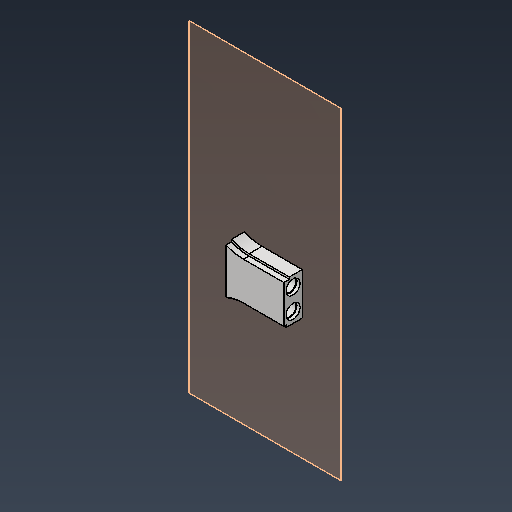
# Autodesk Inventor part: BearigHold
Saved by Autodesk Inventor 2026.2 (Build 302298010, 298A)
## iProperties
Created: 2026-04-04
Part Number: BearigHold
Material: Generic
Document SubType Name: Modeling
Designer: szymo
Density: 1 g/cm^3
Appearance: Default
Author: szymo
Autodesk Inventor part; units mm, degrees
ref_plane "YZ Plane" through (0, 0, 0) normal (1, 0, 0) x (0, 1, 0)
ref_plane "XZ Plane" through (0, 0, 0) normal (0, 1, 0) x (-1, 0, 0)
ref_plane "XY Plane" through (0, 0, 0) normal (0, 0, 1) x (1, 0, 0)
ref_plane "Work Plane1" through (11.7, -32.6479, 0) normal (0, 0, 1) x (-1, 0, 0)
sketch "Sketch1" plane through (11.7, -32.6479, 0) normal (0, 0, 1) x (-1, 0, 0)
  circle A0 centre (14.5, -14.5) radius 13.85 projected
  circle A1 centre (14.5, -14.5) radius 14.5 projected
  circle A2 centre (14.5, -55.2958) radius 13.85 projected
  circle A3 centre (14.5, -55.2958) radius 14.5 projected
  circle A4 centre (13, -35.0012) radius 5 projected
  line L0 (0, 0) -> (33.1738, 0)
  line L1 (33.1738, 0) -> (33.1738, -67)
  line L2 (33.1738, -67) -> (0, -67)
  line L3 (0, -67) -> (0, 0)
  line L4 (2, 0) -> (2, -67)
  line L5 (14.5, -28.35) -> (2, -28.35)
  line L6 (14.5, -29) -> (2, -29)
  line L7 (14.5, -40.7958) -> (2, -40.7958)
  line L8 (14.5, -41.4458) -> (2, -41.4458)
  line L9 (20, 0) -> (20, -67)
  point P0 (11.7, -32.6479)
  point P1 (20, -42.5847)
  point P2 (20, -27.2111)
  point P3 (20, -41.8794)
  point P4 (20, -27.9164)
  dimension "d0" = 67
  dimension "d1" = 2
  dimension "d2" = 2
  constraints: 20 end point, 8 point on line, 7 perpendicular, 5 horizontal, 2 parallel, 1 coincident, 9 other
  measures "d0" distance of L2.end L0.start
  measures "d1" distance between parallel lines of L4 L3
  measures "d2" distance edge to line of A4 L9
ref_plane "Work Plane2" through (-23.2799, 2.168, 4) normal (0, 0, -1) x (-0.6704745, 0.7419326, 0)
extrude "Extrusion1" add sketch "Sketch1" along normal up to surface (4 mm away) contours L9 A1 L5 A0 | L9 A3 L7 L4 L6 A1 | A1 L6 L4 L5 | L9 A2 L8 A3 | A3 L8 L4 L7
ref_plane "Work Plane3" through (-21.8144, -37.1623, 4.9) normal (0, 0, -1) x (-0.3909035, 0.9204317, 0)
extrude "Extrusion2" add sketch "Sketch1" along normal up to surface (4.9 mm away) contours L9 A1 L5 A0 | L9 A3 L7 L4 L6 A1 | A1 L6 L4 L5
extrude "Extrusion3" add sketch "Sketch1" along normal blind 5.3 contours L9 A3 L7 L4 L6 A1
sketch "Sketch2" plane through (11.7, -32.6479, 5.3) normal (0, 0, 1) x (1, 0, 0)
  arc A0 (-14.5, 29) -> (-20, 27.9164) centre (-14.5, 14.5) ccw projected
  line L0 (-14.5, 29) -> (-2, 29) projected
  line L1 (-2, 29) -> (-2, 40.7958) projected
  line L2 (-2, 40.7958) -> (-14.5, 40.7958) projected
  arc A1 (-20, 41.8794) -> (-14.5, 40.7958) centre (-14.5, 55.2958) ccw projected
  line L3 (-20, 41.8794) -> (-20, 27.9164) projected
  circle A2 centre (-13, 35.0012) radius 5 projected
  point P0 (-11.7, 32.6479)
extrude "Extrusion4" add sketch "Sketch2" along normal blind 0.4 contours A0 L3 A1 L2 L1 L0 | A2
sketch "Sketch3" plane through (9.7, -4.2979, 0) normal (1, 0, 0) x (0, 0, -1)
  line L0 (-4.9, 0) -> (-4.9, 0.65) projected
  line L1 (0, 0) -> (-4.9, 0) projected
  line L2 (0, 0) -> (0, 13.0958) projected
  line L3 (0, 13.0958) -> (-4, 13.0958) projected
  line L4 (-4, 12.4458) -> (-4, 13.0958) projected
  line L5 (-4, 12.4458) -> (-5.7, 12.4458) projected
  line L6 (-5.7, 0.65) -> (-5.7, 12.4458) projected
  line L7 (-4.9, 0.65) -> (-5.7, 0.65) projected
  line L8 (-5.7, 6.5479) -> (0, 6.5479)
  line L9 (-5.7, 6.5479) -> (0, 0)
  line L10 (-5.7, 6.5479) -> (0, 13.0958)
  line L11 (0, 6.5479) -> (-2.85, 9.8219)
  line L12 (0, 6.5479) -> (-2.85, 3.274)
  point P0 (0, 4.2979)
  dimension "d11" = 6.5479
  dimension "d12" = 6.5479
  constraints: 10 end point, 4 midpoint, 2 coincident, 1 perpendicular
  measures "d11" distance between parallel lines of L1 L8
  measures "d12" distance between parallel lines of L3 L8
hole "Hole1" at (9.7, -1.024, 2.85) at (9.7, 5.524, 2.85) direction (-1, 0, 0) diameter 4 depth 5.5 counterbore diameter 4.5 counterbore depth 1
equation "\"d11\" = d12"
body "Solid1"
